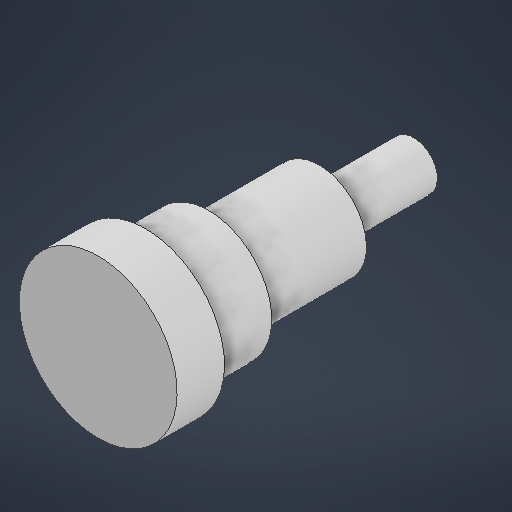
# Autodesk Inventor part: Part2
Saved by Autodesk Inventor 2026 (Build 300175050, 175E)
## iProperties
Created: 2026-03-26
Part Number: Part2
Material: Generic
Document SubType Name: Modeling
Designer: Administrator
Density: 1 g/cm^3
Appearance: Default
Author: Administrator
Autodesk Inventor part; units mm, degrees
ref_plane "YZ Plane" through (0, 0, 0) normal (1, 0, 0) x (0, 1, 0)
ref_plane "XZ Plane" through (0, 0, 0) normal (0, 1, 0) x (-1, 0, 0)
ref_plane "XY Plane" through (0, 0, 0) normal (0, 0, 1) x (1, 0, 0)
sketch "Sketch1" plane through (0, 0, 0) normal (1, 0, 0) x (0, 1, 0)
  line L0 (0, 0) -> (0, -100)
  line L1 (0, -100) -> (7.5, -100)
  line L2 (7.5, -100) -> (7.5, -70)
  line L3 (7.5, -70) -> (15, -70)
  line L4 (15, -70) -> (15, -35)
  line L5 (15, -35) -> (20, -35)
  line L6 (20, -35) -> (20, -15)
  line L7 (20, -15) -> (25, -15)
  line L8 (25, -15) -> (25, 0)
  line L9 (25, 0) -> (0, 0)
  dimension "d0" = 100
  dimension "d1" = 15
  dimension "d2" = 20
  dimension "d3" = 35
  dimension "d4" = 15
  dimension "d5" = 30
  dimension "d6" = 40
  dimension "d7" = 50
  constraints: 20 end point, 6 perpendicular, 3 vertical, 1 horizontal
  measures "d0" distance of L0.start L0.end
  measures "d1" distance of L7.end L8.end
  measures "d2" distance of L5.end L6.end
  measures "d3" distance of L3.end L4.end
  measures "d4" diameter of L2 L0
  measures "d5" diameter of L4 L0
  measures "d6" diameter of L6 L0
  measures "d7" diameter of L8 L0
revolve "Revolution1" add sketch "Sketch1" angle 360 mid plane about axis through (0, 0, 0) along (0, 0, -1)
body "Solid1"
